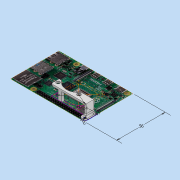
# Autodesk Inventor part: raspberry_fan_holder
Saved by Autodesk Inventor 2022 (Build 260153000, 153)
## iProperties
Created: 2022-08-22
Part Number: raspberry_fan_holder
Material: Générique
Document SubType Name: Modeling
Designer: andre
Density: 1 g/cm^3
Appearance: Par défaut
Author: andre
Autodesk Inventor part; units mm, degrees
ref_plane "YZ Plane" through (0, 0, 0) normal (1, 0, 0) x (0, 1, 0)
ref_plane "XZ Plane" through (0, 0, 0) normal (0, 1, 0) x (-1, 0, 0)
ref_plane "XY Plane" through (0, 0, 0) normal (0, 0, 1) x (1, 0, 0)
sketch "Esquisse1" plane through (0, 0, 0) normal (0, 1, 0) x (-1, 0, 0)
  line L0 (-3.2157, 3.3261) -> (82.1119, 3.3261) construction
  line L1 (82.1119, 3.3261) -> (82.1119, -52.6739) construction
  line L2 (82.1119, -52.6739) -> (-3.2157, -52.6739) construction
  line L3 (-3.2157, -52.6739) -> (-3.2157, 3.3261) construction
  circle A0 centre (0, 0) radius 1.5
  circle A1 centre (0, 0) radius 3
  line L4 (3, 0) -> (3, -3.0737)
  line L5 (-3, 0) -> (-3, -11.6349)
  line L6 (-3, -11.6349) -> (14.9617, -11.6349)
  line L7 (41.5449, -5.1055) -> (11.5449, -5.1055) construction
  line L8 (11.5449, -5.1055) -> (11.5449, -35.1055) construction
  line L9 (11.5449, -35.1055) -> (41.5449, -35.1055) construction
  line L10 (41.5449, -35.1055) -> (41.5449, -5.1055) construction
  line L11 (41.5449, -5.1055) -> (11.5449, -35.1055) construction
  line L12 (11.5449, -5.1055) -> (41.5449, -35.1055) construction
  line L13 (14.5449, -8.1055) -> (38.5449, -8.1055) construction
  line L14 (38.5449, -8.1055) -> (38.5449, -32.1055) construction
  line L15 (38.5449, -32.1055) -> (14.5449, -32.1055) construction
  line L16 (14.5449, -32.1055) -> (14.5449, -8.1055) construction
  line L17 (14.5449, -8.1055) -> (38.5449, -32.1055) construction
  line L18 (38.5449, -8.1055) -> (14.5449, -32.1055) construction
  circle A2 centre (38.5449, -8.1055) radius 2
  circle A3 centre (14.5449, -8.1055) radius 2
  circle A4 centre (14.5449, -32.1055) radius 2 construction
  circle A5 centre (38.5449, -32.1055) radius 2 construction
  circle A6 centre (26.5449, -20.1055) radius 14.35 construction
  arc A7 (38.5449, -12.2364) -> (14.9617, -11.6349) centre (26.5449, -20.1055) ccw
  line L19 (38.5449, -12.2364) -> (41.5449, -12.2364)
  line L20 (41.5449, -12.2364) -> (41.5449, -3.0737)
  line L21 (41.5449, -3.0737) -> (3, -3.0737)
  line L22 (3, -3.0737) -> (3, -11.6349)
  dimension "d1" = 56
  dimension "d9" = 3
  dimension "d10" = 6
  dimension "d20" = 30
  dimension "d21" = 24
  dimension "d22" = 4
  dimension "d23" = 4
  dimension "d24" = 4
  dimension "d25" = 4
  dimension "d34" = 28.7
  constraints: 38 end point, 8 centre point, 8 perpendicular, 7 coincident, 6 point on circle, 5 parallel, 4 midpoint, 4 point on line, 2 horizontal, 2 tangent, 1 concentric, 1 vertical, 2 other
  measures "d1" distance of L2.end L0.start
  measures "d9" diameter of A0
  measures "d10" diameter of A1
  measures "d20" distance of L8.end L9.end
  measures "d21" distance of L14.end L15.end
  measures "d22" diameter of A2
  measures "d23" diameter of A5
  measures "d24" diameter of A4
  measures "d25" diameter of A3
  measures "d34" diameter of A6
extrude "Extrusion3" add sketch "Esquisse1" along normal blind 1.5 contours A1 | L4 L22 L6 L5 A1
sketch "Esquisse3" plane through (0, 1.5, 0) normal (0, 1, 0) x (1, 0, 0)
  line L0 (-41.5449, 3.0737) -> (-3, 3.0737) projected
  line L1 (3, 11.6349) -> (-14.9617, 11.6349) projected
  line L2 (-3, 11.6349) -> (-3, 0) projected
  line L3 (3, 11.6349) -> (-3, 11.6349) projected
  line L4 (-3, 3.0737) -> (-1, 3.0737)
  line L5 (-1, 3.0737) -> (-1, 11.6349)
  line L6 (-1, 11.6349) -> (-3, 11.6349)
  line L7 (-3, 11.6349) -> (-3, 3.0737)
  point P0 (0, 0)
  dimension "d59" = 2
  constraints: 8 end point, 2 parallel, 1 horizontal, 1 perpendicular, 1 point on line
  measures "d59" distance of L0.end L4.end
extrude "Extrusion4" add sketch "Esquisse3" along normal blind 11
sketch "Esquisse4" plane through (0, 12.5, 0) normal (0, 1, 0) x (1, 0, 0)
  line L0 (3, 11.6349) -> (-14.9617, 11.6349) projected
  line L1 (-41.5449, 3.0737) -> (-3, 3.0737) projected
  circle A0 centre (-14.5449, 8.1055) radius 2 projected
  arc A1 (-38.5449, 12.2364) -> (-14.9617, 11.6349) centre (-26.5449, 20.1055) ccw projected
  circle A2 centre (-38.5449, 8.1055) radius 2 projected
  line L2 (-38.5449, 12.2364) -> (-41.5449, 12.2364) projected
  line L3 (-41.5449, 12.2364) -> (-41.5449, 3.0737)
  line L4 (3, 11.6349) -> (-3, 11.6349) projected
  line L5 (-1, 3.0737) -> (-3, 3.0737) projected
  line L6 (-3, 11.6349) -> (-3, 3.0737)
  point P0 (0, 0)
  constraints: 4 end point, 2 vertical
extrude "Extrusion5" add sketch "Esquisse4" against normal blind 2
sketch "Esquisse5" plane through (0, 10.5, 0) normal (0, -1, 0) x (1, 0, 0)
  line L0 (-41.5449, -3.0737) -> (-1, -3.0737) projected
  line L1 (-33.5622, -3.0737) -> (-33.5622, -7.6396)
  line L2 (-29.4015, -3.0737) -> (-29.4015, -6.0427)
  arc A0 (-14.9617, -11.6349) -> (-38.5449, -12.2364) centre (-26.5449, -20.1055) ccw projected
  arc A1 (-29.4015, -6.0427) -> (-33.5622, -7.6396) centre (-26.909, -18.7556) ccw
  line L3 (-33.5622, -3.0737) -> (-29.4015, -3.0737)
  point P0 (0, 0)
  point P1 (-31.1473, -6.5135)
  point P2 (-33.5622, -7.5883)
  constraints: 6 end point, 3 point on circle, 2 point on line, 2 vertical, 1 centre point, 1 perpendicular
extrude "Extrusion6" add sketch "Esquisse5" along normal blind 11.3 contours L0 L2 A1 A0 L1
fillet "Congé3" radius 3 1 edges at (3, 0.75, -11.6349)
fillet "Congé4" radius 1 2 edges at (-1, 1.5, -7.3543) (-2, 1.5, -3.0737)
fillet "Congé5" radius 2 1 edges at (-41.5449, 11.5, -3.0737)
equation "\"d23\" = d22"
equation "\"d24\" = d22"
equation "\"d25\" = d22"
